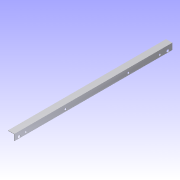
# Autodesk Inventor part: GE-09031-01
Saved by Autodesk Inventor 2012 (Build 160160000, 160)
## iProperties
Created: 2008-05-27
Part Number: GE-09031-01
Description: Upper Rail
Document SubType Name: Modeling
Designer: narosenberg
Density: 1 g/cm^3
Material: Default
Author: dfoster
Autodesk Inventor part; units mm, degrees
ref_plane "YZ Plane" through (0, 0, 0) normal (1, 0, 0) x (0, 1, 0)
ref_plane "XZ Plane" through (0, 0, 0) normal (0, 1, 0) x (-1, 0, 0)
ref_plane "XY Plane" through (0, 0, 0) normal (0, 0, 1) x (1, 0, 0)
sketch "Sketch1" plane through (0, 0, 0) normal (0, 0, 1) x (1, 0, 0)
  line L0 (-21.1568, 46.0602) -> (29.6432, 46.0602)
  line L1 (29.6432, 46.0602) -> (29.6432, -4.7398)
  line L2 (29.6432, -4.7398) -> (26.4682, -4.7398)
  line L3 (-21.1568, 42.8852) -> (-21.1568, 46.0602)
  line L4 (-21.1568, 42.8852) -> (26.4682, 42.8852)
  line L5 (26.4682, 42.8852) -> (26.4682, -4.7398)
  dimension "d0" = 50.8
  dimension "d1" = 50.8
  dimension "d2" = 3.175
  dimension "d3" = 3.175
  constraints: 12 end point, 2 horizontal, 2 parallel, 2 perpendicular
  measures "d0" distance of L0.start L0.end
  measures "d1" distance of L0.end L1.end
  measures "d2" distance between parallel lines of L0 L4
  measures "d3" distance between parallel lines of L1 L5
extrude "Extrusion1" add sketch "Sketch1" along normal blind 1274.7625
sketch "Sketch2" plane through (26.4682, -4.7398, 0) normal (-1, 0, 0) x (0, 0, 1)
  circle A0 centre (36.5125, 12.7) radius 10.3188
  line L0 (0, 50.8) -> (1274.7625, 50.8) projected
  circle A1 centre (100.0125, 17.4625) radius 7.1437
  circle A2 centre (354.0125, 17.4625) radius 7.1437
  circle A3 centre (862.0125, 17.4625) radius 7.1437
  circle A4 centre (1181.1, 17.4625) radius 7.1437
  circle A5 centre (1236.6625, 12.7) radius 10.3188
  line L1 (1274.7625, 0) -> (1274.7625, 47.625) projected
  dimension "d8" = 20.6375
  dimension "d12" = 38.1
  dimension "d14" = 14.2875
  dimension "d15" = 14.2875
  dimension "d16" = 14.2875
  dimension "d17" = 14.2875
  dimension "d25" = 20.6375
  dimension "d26" = 38.1
  dimension "d27" = 38.1
  dimension "d28" = 93.6625
  dimension "d29" = 412.75
  dimension "d30" = 920.75
  dimension "d31" = 1174.75
  dimension "d33" = 1238.25
  dimension "d34" = 33.3375
  constraints: 6 centre point, 3 horizontal alignment
  measures "d8" diameter of A0
  measures "d12" distance from line of A0.centre L0
  measures "d14" diameter of A1
  measures "d15" diameter of A2
  measures "d16" diameter of A3
  measures "d17" diameter of A4
  measures "d25" diameter of A5
  measures "d26" distance from line of L0 A5.centre
  measures "d27" distance from line of A5.centre L1
  measures "d28" distance from line of A4.centre L1
  measures "d29" distance from line of A3.centre L1
  measures "d30" distance from line of A2.centre L1
  measures "d31" distance from line of A1.centre L1
  measures "d33" distance from line of A0.centre L1
  measures "d34" distance from line of L0 A4.centre
extrude "Extrusion2" cut sketch "Sketch2" against normal blind 1812.925
equation "\"d15\" = d14"
equation "\"d16\" = d14"
equation "\"d17\" = d14"
equation "\"d25\" = d8"
equation "\"d26\" = d12"
body "Solid1"
